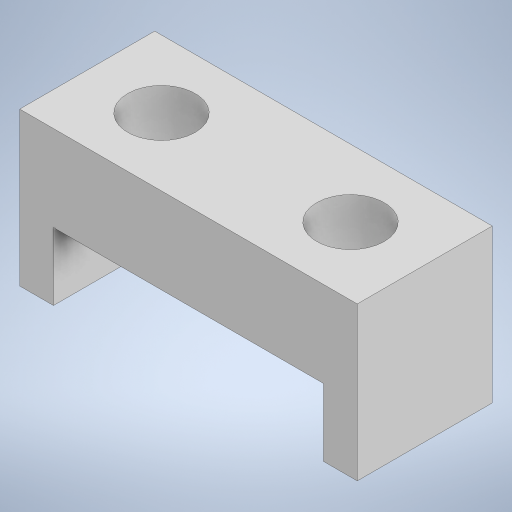
# Autodesk Inventor part: Idle Bearing mount
Saved by Autodesk Inventor 2023.1 (Build 271208000, 208)
## iProperties
Created: 2022-10-29
Part Number: Idle Bearing mount
Material: Generic
Document SubType Name: Modeling
Designer: nicol
Density: 1 g/cm^3
Appearance: Default
Author: nicol
Autodesk Inventor part; units mm, degrees
ref_plane "YZ Plane" through (0, 0, 0) normal (1, 0, 0) x (0, 1, 0)
ref_plane "XZ Plane" through (0, 0, 0) normal (0, 1, 0) x (-1, 0, 0)
ref_plane "XY Plane" through (0, 0, 0) normal (0, 0, 1) x (1, 0, 0)
sketch "Sketch1" plane through (0, 0, 0) normal (0, 0, 1) x (1, 0, 0)
  line L0 (0, 0) -> (25, 0)
  line L1 (25, 0) -> (25, 6.35)
  line L2 (25, 6.35) -> (0, 6.35)
  line L3 (0, 6.35) -> (0, 0)
  line L4 (0, 0) -> (0, -5)
  line L5 (0, -5) -> (2.5, -5)
  line L6 (2.5, -5) -> (2.5, 0)
  line L7 (25, 0) -> (25, -5)
  line L8 (25, -5) -> (22.5, -5)
  line L9 (22.5, -5) -> (22.5, 0)
  dimension "d0" = 25
  dimension "d1" = 6.35
  dimension "d14" = 20
  dimension "d15" = 5
  constraints: 20 end point, 6 perpendicular, 2 equal length, 2 parallel, 2 point on line, 1 horizontal, 1 vertical
  measures "d0" distance of L1.end L2.end
  measures "d1" distance of L0.end L1.end
  measures "d14" distance between parallel lines of L6 L9
  measures "d15" distance of L5.end L6.end
extrude "Extrusion1" add sketch "Sketch1" along normal blind 10
sketch "Sketch2" plane through (0, 6.35, 0) normal (0, 1, 0) x (1, 0, 0)
  line L0 (0, 0) -> (0, -10) projected
  line L1 (25, 0) -> (25, -10) projected
  point P0 (5.5, -5)
  point P1 (19.5, -5)
  point P2 (0, -5)
  dimension "d4" = 5.5
  dimension "d5" = 5.5
  dimension "d6" = 14
  constraints: 2 horizontal alignment, 1 midpoint
  measures "d4" distance from line of L1 point (19.5, -5)
  measures "d5" distance from line of point (5.5, -5) L0
  measures "d6" distance of point (5.5, -5) point (19.5, -5)
hole "Hole1" at (5.5, 6.35, 5) at (19.5, 6.35, 5) direction (0, -1, 0) diameter 5 end through all
equation "\"d5\" = d4"
body "Solid1"
